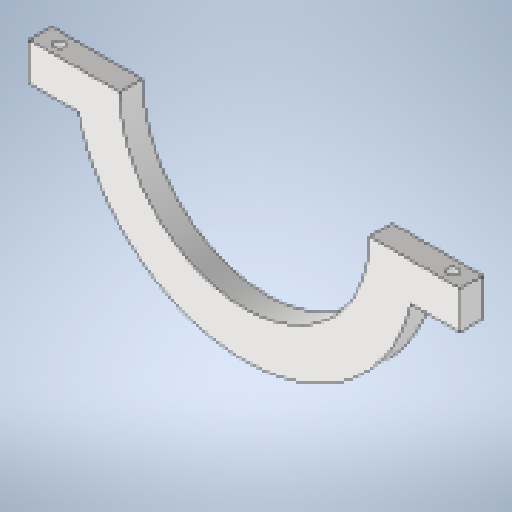
# Autodesk Inventor part: ДМФ 091 Постель НОС v2.0
Saved by Autodesk Inventor 2025.3 (Build 293356030, 356C)
## iProperties
Created: 2024-04-28
Part Number: ДМФ 091 Постель НОС v2.0
Material: Generic
Document SubType Name: Sheet Metal
Designer: admin
Density: 1 g/cm^3
Appearance: Default
Stock Number: Постель_Нос
Flat Pattern Width: 22.5 cm
Flat Pattern Length: 57 cm
Flat Pattern Area: 1282.5 cm^2
Sheet Metal Rule: Default
Sheet Metal Width: 225,000 mm
Sheet Metal Length: 570,000 mm
Sheet Metal Area: 128250,000 mm^2
Author: pokla
Autodesk Inventor part; units mm, degrees
ref_plane "YZ Plane" through (0, 0, 0) normal (1, 0, 0) x (0, 1, 0)
ref_plane "XZ Plane" through (0, 0, 0) normal (0, 1, 0) x (-1, 0, 0)
ref_plane "XY Plane" through (0, 0, 0) normal (0, 0, 1) x (1, 0, 0)
sketch "Sketch1" plane through (0, 0, 0) normal (0, 0, 1) x (1, 0, 0)
  circle A0 centre (0, 0) radius 195 construction
  line L0 (0, 195) -> (0, 225) construction
  line L1 (0, 195) -> (0, 165) construction
  circle A1 centre (0, 0) radius 165
  circle A2 centre (0, 0) radius 225
  line L2 (-225, 0) -> (-165, 0)
  line L3 (165, 0) -> (225, 0)
  line L4 (-225, 0) -> (-285, 0)
  line L5 (-285, 0) -> (-285, -50)
  line L6 (-285, -50) -> (-219.3741, -50)
  line L7 (225, 0) -> (285, 0)
  line L8 (285, 0) -> (285, -50)
  line L9 (285, -50) -> (219.3741, -50)
  line L10 (-32.9068, -209.6114) -> (28.3831, -209.6114)
  line L11 (28.3831, -209.6114) -> (28.3831, -281.9335)
  line L12 (28.3831, -281.9335) -> (-32.9068, -281.9335)
  line L13 (-32.9068, -281.9335) -> (-32.9068, -209.6114)
  dimension "d13" = 390
  dimension "d36" = 60
  dimension "d40" = 60
  dimension "d41" = 50
  constraints: 28 end point, 8 point on circle, 5 perpendicular, 4 horizontal, 3 coincident, 3 equal length, 2 centre point, 2 horizontal alignment, 2 parallel, 2 vertical, 1 line through centre, 1 point on line, 1 vertical alignment, 2 other
  measures "d36" distance of L1.end L0.end
  measures "d40" distance of L2.start L4.end
  measures "d41" distance of L4.end L5.end
extrude "Extrusion1" add sketch "Sketch1" against normal blind 30 contours L3 A2 L11 L10 L13 L2 A1 | L7 L8 L9 A2 | A2 L6 L5 L4 | A2 L13 L10 L11
sketch "Sketch7" plane through (-285, 0, 0) normal (0, 1, 0) x (1, 0, 0)
  circle A0 centre (25, 15) radius 7
  line L0 (0, 0) -> (0, 30) projected
  point P0 (285, 0)
  point P1 (0, 15)
  dimension "d42" = 14
  dimension "d43" = 25
  constraints: 1 centre point, 1 horizontal alignment, 1 midpoint
  measures "d42" diameter of A0
  measures "d43" distance from line of L0 A0.centre
extrude "Extrusion7" cut sketch "Sketch7" against normal through all
mirror "Mirror1" about plane through (0, 0, 0) normal (1, 0, 0) of "Extrusion7"
equation "\"d13\" = Шпил_пласт_НОС_диам_центров"
equation "\"d40\" = d36"
equation "\"BendReliefDepth\" = 0.5 * Thickness"
equation "\"Шпил_пласт_НОС_диам_центров\" = 390"
equation "\"Thickness\" = 30"
body "Solid1"
